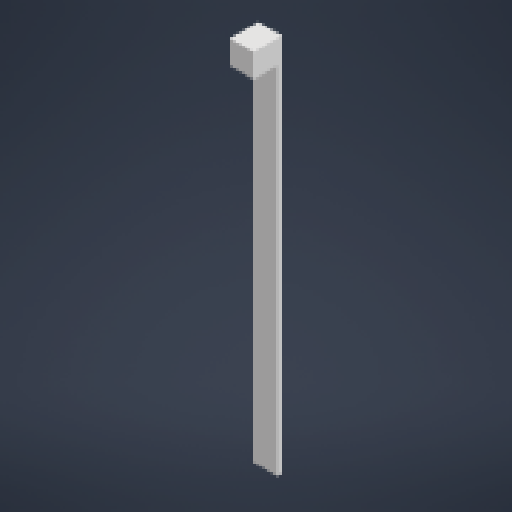
# Autodesk Inventor part: display lock pin
Saved by Autodesk Inventor 2024 (Build 280153000, 153)
## iProperties
Created: 2023-07-17
Part Number: display lock pin
Material: 일반
Document SubType Name: Modeling
Designer: wodyd
Density: 1 g/cm^3
Appearance: 기본값
Author: wodyd
Autodesk Inventor part; units mm, degrees
ref_plane "YZ Plane" through (0, 0, 0) normal (1, 0, 0) x (0, 1, 0)
ref_plane "XZ Plane" through (0, 0, 0) normal (0, 1, 0) x (-1, 0, 0)
ref_plane "XY Plane" through (0, 0, 0) normal (0, 0, 1) x (1, 0, 0)
sketch "스케치1" plane through (0, 0, 0) normal (0, 0, 1) x (1, 0, 0)
  line L0 (-69.2252, 42.3816) -> (-64.2252, 42.3816)
  line L1 (-64.2252, 42.3816) -> (-64.2252, -37.6184)
  line L2 (-64.2252, -37.6184) -> (-69.2252, -37.6184)
  line L3 (-69.2252, -37.6184) -> (-69.2252, 42.3816)
  point P0 (0, 0)
  point P1 (-66.7252, 42.3816)
  dimension "d0" = 5
  dimension "d1" = 80
  constraints: 8 end point, 2 parallel, 1 horizontal, 1 midpoint, 1 perpendicular
  measures "d0" distance of L1.end L2.end
  measures "d1" distance of L0.end L1.end
extrude "돌출1" add sketch "스케치1" along normal blind 1
sketch "스케치2" plane through (0, 0, 1) normal (0, 0, 1) x (1, 0, 0)
  line L0 (-64.2252, 42.3816) -> (-69.2252, 42.3816) projected
  line L1 (-69.2252, 42.3816) -> (-64.2252, 42.3816)
  line L2 (-64.2252, 42.3816) -> (-64.2252, 37.3816)
  line L3 (-64.2252, 37.3816) -> (-69.2252, 37.3816)
  line L4 (-69.2252, 37.3816) -> (-69.2252, 42.3816)
  point P0 (0, 0)
  dimension "d7" = 5
  dimension "d8" = 5
  constraints: 8 end point, 2 parallel, 1 horizontal, 1 perpendicular
  measures "d7" distance of L2.end L3.end
  measures "d8" distance of L1.end L2.end
extrude "돌출2" add sketch "스케치2" along normal blind 5
